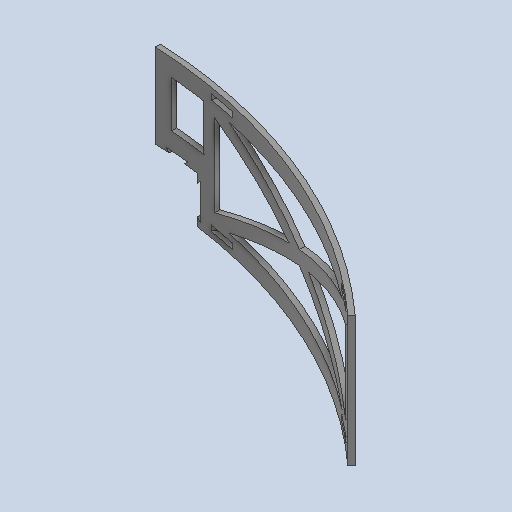
# Autodesk Inventor part: Battery Module Third Iteration Outer Wall
Saved by Autodesk Inventor 2023 (Build 270158000, 158)
## iProperties
Created: 2023-03-05
Part Number: Battery Module Third Iteration Outer Wall
Material: PLA Plastic
Document SubType Name: Modeling
Designer: mihal
Density: 1.25002 g/cm^3
Appearance: Generic
Mass: 30.2461 g
Surface Area: 215.652 cm^2
Volume: 24.1964 cm^3
Author: mihal
Autodesk Inventor part; units mm, degrees
ref_plane "YZ Plane" through (0, 0, 0) normal (1, 0, 0) x (0, 1, 0)
sketch "Sketch1" plane through (0, 0, 0) normal (0, 1, 0) x (-1, 0, 0)
  circle A0 centre (0, 0) radius 215
  circle A1 centre (0, 0) radius 315
  line L0 (0, 0) -> (0, -315)
  line L1 (0, 0) -> (-222.7386, -222.7386)
  line L2 (-141.0509, -162.2641) -> (-211.8794, -233.0926)
  line L3 (-15, -214.4761) -> (-15, -314.6427)
  circle A2 centre (0, 0) radius 219.5
  circle A3 centre (0, 0) radius 310.5
  circle A4 centre (0, 0) radius 222.5
  circle A5 centre (0, 0) radius 307.5
  point P0 (-152.028, -152.028)
  point P1 (0, -215)
  point P2 (0, -312.5)
  point P3 (0, -217.5)
  point P4 (-153.7957, -153.7957)
  point P5 (-220.9709, -220.9709)
  point P6 (-210.1096, -231.3228)
  point P7 (-15, -312.1398)
  point P8 (-15, -216.9821)
  point P9 (-142.8229, -164.0361)
  point P10 (-207.7734, -228.9866)
  point P11 (-15, -308.8359)
  point P12 (-15, -220.2899)
  point P13 (-145.1619, -166.3751)
  point P14 (-15, -310.1375)
  point P15 (-208.6937, -229.9069)
  point P16 (-15, -218.9869)
  point P17 (-144.2405, -165.4537)
  point P18 (-15, -307.1339)
  point P19 (-206.5699, -227.7831)
  dimension "d0" = 430
  dimension "d1" = 630
  dimension "d2" = 45
  dimension "d3" = 15
  dimension "d4" = 15
  dimension "d5" = 4.5
  dimension "d6" = 4.5
  dimension "d20" = 3
  dimension "d21" = 3
  constraints: 8 end point, 6 centre point, 6 coincident, 6 point on circle, 2 parallel, 1 vertical
  measures "d0" diameter of A0
  measures "d1" diameter of A1
  measures "d2" angle of L1 L0
  measures "d3" distance between parallel lines of L2 L1
  measures "d4" distance between parallel lines of L3 L0
  measures "d5" radial gap between concentric circles of A0 A2
  measures "d6" radial gap between concentric circles of A3 A1
  measures "d20" radial gap between concentric circles of A2 A4
  measures "d21" radial gap between concentric circles of A5 A3
extrude "Extrusion1" add sketch "Sketch1" along normal blind 76 contours A5 L3 A3 L2
sketch "Sketch4" plane through (0, 0, 0) normal (0, 0, 1) x (1, 0, 0)
  line L0 (15, 0) -> (206.5699, 0) projected
  line L1 (206.5699, 0) -> (206.5699, 76) projected
  line L2 (15, 76) -> (206.5699, 76) projected
  line L3 (15, 0) -> (15, 76) projected
  line L4 (208.6937, 0) -> (15, 0) projected
  line L5 (15, 0) -> (42, 0)
  line L6 (42, 0) -> (42, 27)
  line L7 (42, 27) -> (15, 27)
  line L8 (15, 27) -> (15, 0)
  line L9 (15, 0) -> (42, 0)
  line L10 (42, 0) -> (42, 27)
  line L11 (42, 27) -> (15, 27)
  line L12 (15, 27) -> (15, 0)
  line L13 (42, 5) -> (44, 3)
  line L14 (44, 3) -> (44, 24)
  line L15 (44, 24) -> (42, 22)
  line L16 (23.5, 27) -> (21.5, 29)
  line L17 (21.5, 29) -> (35.5, 29)
  line L18 (35.5, 29) -> (33.5, 27)
  point P0 (0, 0)
  dimension "d22" = 27
  dimension "d23" = 27
  dimension "d26" = 27
  dimension "d27" = 27
  dimension "d28" = 2
  dimension "d29" = 2
  dimension "d30" = 2
  dimension "d31" = 21
  dimension "d32" = 2
  dimension "d33" = 2
  dimension "d34" = 2
  dimension "d35" = 6.5
  dimension "d36" = 6.5
  constraints: 28 end point, 5 parallel, 4 point on line, 3 horizontal, 2 perpendicular
  measures "d22" distance of L7.end L6.end
  measures "d23" distance of L6.end L5.end
  measures "d26" distance of L11.end L10.end
  measures "d27" distance of L10.end L9.end
  measures "d28" distance between parallel lines of L10 L14
  measures "d29" horizontal distance of L14.end L15.end
  measures "d30" horizontal distance of L13.end L13.start
  measures "d31" distance of L13.end L14.end
  measures "d32" distance between parallel lines of L11 L17
  measures "d33" horizontal distance of L16.end L16.start
  measures "d34" horizontal distance of L17.end L18.end
  measures "d35" horizontal distance of L11.end L16.end
  measures "d36" horizontal distance of L10.end L17.end
extrude "Extrusion4" cut sketch "Sketch4" against normal up to surface contours L3 L7 L6 L0 | L6 L15 L14 L13 | L16 L17 L18 L7 round surface about axis through (0, 0, 0) along (0, 1, 0) radius 310.5 far side no
sketch "Sketch8" plane through (0, 0, 0) normal (0, 0, 1) x (1, 0, 0)
  line L0 (42, 5) -> (42, 0) projected
  line L1 (42, 0) -> (206.5699, 0) projected
  line L2 (206.5699, 0) -> (206.5699, 76) projected
  line L3 (15, 76) -> (206.5699, 76) projected
  line L4 (15, 27) -> (15, 76) projected
  line L5 (15, 27) -> (23.5, 27) projected
  line L6 (23.5, 27) -> (21.5, 29) projected
  line L7 (21.5, 29) -> (35.5, 29) projected
  line L8 (35.5, 29) -> (33.5, 27) projected
  line L9 (33.5, 27) -> (42, 27) projected
  line L10 (42, 27) -> (42, 22) projected
  line L11 (42, 22) -> (44, 24) projected
  line L12 (44, 24) -> (44, 3) projected
  line L13 (44, 3) -> (42, 5) projected
  line L14 (15, 27) -> (15, 76) projected
  line L15 (15, 39) -> (54, 39)
  line L16 (54, 39) -> (54, 0)
  line L17 (25, 39) -> (25, 66)
  line L18 (25, 66) -> (196.5699, 66)
  line L19 (196.5699, 66) -> (196.5699, 10)
  line L20 (196.5699, 10) -> (54, 10)
  line L21 (54, 39) -> (54, 66)
  line L22 (46.5, 39) -> (46.5, 66)
  line L23 (54, 66) -> (196.5699, 10) construction
  line L24 (54, 10) -> (196.5699, 66) construction
  line L25 (64.2572, 66) -> (196.5699, 14.0289)
  line L26 (54, 61.9711) -> (186.3127, 10)
  line L27 (54, 14.0289) -> (186.3127, 66)
  line L28 (64.2572, 10) -> (196.5699, 61.9711)
  point P0 (0, 0)
  point P1 (15, 51.5)
  point P2 (135.5421, 38)
  point P3 (125.2849, 33.9711)
  point P4 (125.2849, 42.0289)
  point P5 (115.0278, 38)
  dimension "d119" = 10
  dimension "d120" = 10
  dimension "d121" = 10
  dimension "d122" = 10
  dimension "d123" = 10
  dimension "d124" = 10
  dimension "d125" = 7.5
  dimension "d126" = 7.5
  dimension "d127" = 7.5
  constraints: 28 end point, 15 point on line, 6 perpendicular, 4 parallel, 1 horizontal, 1 midpoint, 1 vertical, 2 other
  measures "d119" distance between parallel lines of L7 L15
  measures "d120" distance from line of point (15, 51.5) L17
  measures "d121" distance between parallel lines of L3 L18
  measures "d122" distance between parallel lines of L12 L16
  measures "d123" distance between parallel lines of L1 L20
  measures "d124" distance between parallel lines of L2 L19
  measures "d125" distance between parallel lines of L21 L22
  measures "d126" distance between parallel lines of L26 L25
  measures "d127" distance between parallel lines of L28 L27
extrude "Extrusion8" cut sketch "Sketch8" against normal up to surface contours L16 L21 L26 L27 | L28 L26 L20 | L15 L17 L18 L22 | L25 L18 L27 | L28 L19 L25 round surface about axis through (0, 0, 0) along (0, 1, 0) radius 310.5 far side no
ref_plane "Work Plane5" through (15, 0, -307.1339) normal (0.3826834, 0, -0.9238795) x (0, 1, 0)
ref_plane "Work Plane6" through (15, 0, -307.1339) normal (0.3826834, 0, -0.9238795) x (0, 1, 0)
sketch "Sketch10" plane through (15, 0, -307.1339) normal (0.3826834, 0, -0.9238795) x (0, 1, 0)
  line L0 (66, 47.9655) -> (66, 182.1915) projected
  ellipse E0 centre (-7.1817, 103.6769) end of major axis (106.5381, 410.8074) minor radius 43.3979 (42.0289, 111.9599) -> (66, 182.1915) ccw projected
  ellipse E1 centre (91.2396, 103.6769) end of major axis (-22.4803, 410.8074) minor radius 43.3979 (42.0289, 111.9599) -> (66, 47.9655) ccw projected
  line L1 (66, 30.3154) -> (39, 30.3154) projected
  line L2 (39, 30.3154) -> (39, 9.4883) projected
  line L3 (39, 9.4883) -> (66, 9.4883) projected
  line L4 (66, 9.4883) -> (66, 30.3154) projected
  ellipse E2 centre (-15.2396, 103.6769) end of major axis (98.4803, 410.8074) minor radius 43.3979 (38, 123.2749) -> (61.9711, 194.7918) ccw projected
  line L5 (61.9711, 194.7918) -> (14.0289, 194.7918) projected
  ellipse E3 centre (91.2396, 103.6769) end of major axis (-22.4803, 410.8074) minor radius 43.3979 (14.0289, 194.7918) -> (38, 123.2749) ccw projected
  ellipse E4 centre (83.1817, 103.6769) end of major axis (-30.5381, 410.8074) minor radius 43.3979 (38, 100.8169) -> (61.9711, 37.7199) ccw projected
  ellipse E5 centre (-7.1817, 103.6769) end of major axis (106.5381, 410.8074) minor radius 43.3979 (14.0289, 37.7199) -> (38, 100.8169) ccw projected
  line L6 (14.0289, 37.7199) -> (61.9711, 37.7199) projected
  ellipse E6 centre (-15.2396, 103.6769) end of major axis (98.4803, 410.8074) minor radius 43.3979 (10, 47.9655) -> (33.9711, 111.9599) ccw projected
  ellipse E7 centre (83.1817, 103.6769) end of major axis (-30.5381, 410.8074) minor radius 43.3979 (10, 182.1915) -> (33.9711, 111.9599) ccw projected
  line L7 (10, 182.1915) -> (10, 47.9655) projected
  line L8 (5, 25.9075) -> (0, 25.9075) projected
  line L9 (0, 25.9075) -> (0, 207.3537) projected
  line L10 (0, 207.3537) -> (76, 207.3537) projected
  line L11 (76, 0) -> (76, 207.3537) projected
  line L12 (27, 0) -> (76, 0) projected
  line L13 (27, 0) -> (27, 8.057) projected
  ellipse E8 centre (50.5, 103.6769) end of major axis (-251.0915, 405.2683) minor radius 84.8391 (27, 8.057) -> (29, 6.1531) ccw projected
  line L14 (29, 6.1531) -> (29, 19.5863) projected
  ellipse E9 centre (-6.5, 103.6769) end of major axis (295.0915, 405.2683) minor radius 84.8391 (27, 17.6521) -> (29, 19.5863) ccw projected
  line L15 (27, 17.6521) -> (27, 25.9075) projected
  line L16 (27, 25.9075) -> (22, 25.9075) projected
  ellipse E10 centre (-20, 103.6769) end of major axis (281.5915, 405.2683) minor radius 84.8391 (22, 25.9075) -> (24, 27.8633) ccw projected
  line L17 (24, 27.8633) -> (3, 27.8633) projected
  ellipse E11 centre (47, 103.6769) end of major axis (-254.5915, 405.2683) minor radius 84.8391 (3, 27.8633) -> (5, 25.9075) ccw projected
  line L18 (61.9711, 37.7199) -> (76, 37.7199) construction
  line L19 (66, 47.9655) -> (76, 47.9655) construction
  line L20 (66, 182.1915) -> (76, 182.1915) construction
  line L21 (61.9711, 194.7918) -> (76, 194.7918) construction
  line L22 (13.5, 37.7199) -> (0, 37.7199) construction
  line L23 (10, 47.9655) -> (0, 47.9655) construction
  line L24 (10, 182.1915) -> (0, 182.1915) construction
  line L25 (14.0289, 194.7918) -> (0, 194.7918) construction
  line L26 (3.2, 207.3537) -> (3.2, 27.7952) construction
  line L27 (72.8, 0) -> (72.8, 207.3537) construction
  line L28 (71, 47.9655) -> (71, 37.7199) construction
  line L29 (71, 182.1915) -> (71, 194.7918) construction
  line L30 (5, 47.9655) -> (5, 37.7199) construction
  line L31 (5, 182.1915) -> (5, 194.7918) construction
  line L32 (5, 42.8427) -> (16.0502, 42.8427) construction
  line L33 (71, 42.8427) -> (59.9498, 42.8427) construction
  line L34 (71, 188.4917) -> (60.4365, 188.4917) construction
  ellipse E12 centre (-15.2396, 103.6769) end of major axis (-130.0689, -206.4501) minor radius 43.8213 (38, 121.9974) -> (61.9711, 193.3039) ccw construction
  line L35 (5, 188.4917) -> (16.0324, 188.4917) construction
  line L36 (6.4, 180.8917) -> (3.2, 180.8917)
  line L37 (3.2, 180.8917) -> (3.2, 196.0917)
  line L38 (3.2, 196.0917) -> (6.4, 196.0917)
  line L39 (6.4, 196.0917) -> (6.4, 180.8917)
  line L40 (6.4, 180.8917) -> (3.2, 196.0917) construction
  line L41 (3.2, 180.8917) -> (6.4, 196.0917) construction
  line L42 (3.2, 35.2427) -> (6.4, 35.2427)
  line L43 (6.4, 35.2427) -> (6.4, 50.4427)
  line L44 (6.4, 50.4427) -> (3.2, 50.4427)
  line L45 (3.2, 50.4427) -> (3.2, 35.2427)
  line L46 (3.2, 35.2427) -> (6.4, 50.4427) construction
  line L47 (6.4, 35.2427) -> (3.2, 50.4427) construction
  line L48 (69.6, 35.2427) -> (72.8, 35.2427)
  line L49 (72.8, 35.2427) -> (72.8, 50.4427)
  line L50 (72.8, 50.4427) -> (69.6, 50.4427)
  line L51 (69.6, 50.4427) -> (69.6, 35.2427)
  line L52 (69.6, 35.2427) -> (72.8, 50.4427) construction
  line L53 (72.8, 35.2427) -> (69.6, 50.4427) construction
  line L54 (69.6, 180.8917) -> (72.8, 180.8917)
  line L55 (72.8, 180.8917) -> (72.8, 196.0917)
  line L56 (72.8, 196.0917) -> (69.6, 196.0917)
  line L57 (69.6, 196.0917) -> (69.6, 180.8917)
  line L58 (69.6, 180.8917) -> (72.8, 196.0917) construction
  line L59 (72.8, 180.8917) -> (69.6, 196.0917) construction
  line L60 (71, 188.4917) -> (72.8, 188.4917) construction
  line L61 (71, 42.8427) -> (72.8, 42.8427) construction
  line L62 (5, 42.8427) -> (3.2, 42.8427) construction
  line L63 (5, 188.4917) -> (3.2, 188.4917) construction
  point P0 (0, 103.6769)
  point P1 (4.8, 188.4917)
  point P2 (4.8, 42.8427)
  point P3 (71.2, 42.8427)
  point P4 (71.2, 188.4917)
  dimension "d140" = 3.2
  dimension "d141" = 3.2
  dimension "d142" = 3.2
  dimension "d143" = 15.2
  dimension "d144" = 15.2
  dimension "d145" = 3.2
  dimension "d146" = 15.2
  dimension "d147" = 3.2
  dimension "d148" = 15.2
  dimension "d149" = 3.2
  constraints: 92 end point, 34 point on line, 20 midpoint, 12 parallel, 10 perpendicular, 6 horizontal, 1 coincident, 1 collinear, 17 other
  measures "d140" distance between parallel lines of L9 L26
  measures "d141" distance between parallel lines of L11 L27
  measures "d142" distance of L37.end L38.end
  measures "d143" distance of L36.end L37.end
  measures "d144" distance of L42.end L43.end
  measures "d145" distance of L43.end L44.end
  measures "d146" distance of L48.end L49.end
  measures "d147" distance of L49.end L50.end
  measures "d148" distance of L54.end L55.end
  measures "d149" distance of L55.end L56.end
extrude "Extrusion10" cut sketch "Sketch10" along normal up to surface contours L36 L37 L38 L39 | L45 L44 L43 L42 | L51 L50 L49 L48 | L57 L56 L55 L54 round surface about axis through (0, 0, 0) along (0, 1, 0) radius 310.5 far side no
equation "\"d141\" = d140"
equation "\"d144\" = d143"
equation "\"d145\" = d142"
equation "\"d146\" = d143"
equation "\"d147\" = d142"
equation "\"d148\" = d143"
equation "\"d149\" = d142"
body "Solid1"
